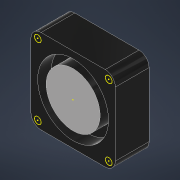
# Autodesk Inventor part: fan
Saved by Autodesk Inventor 2021 (Build 250183000, 183)
## iProperties
Created: 2021-01-23
Part Number: fan
Material: Polyethylene, Low Density
Document SubType Name: Modeling
Designer: User
Density: 0.894 g/cm^3
Appearance: Smooth - Black
Author: User
Autodesk Inventor part; units mm, degrees
ref_plane "YZ Plane" through (0, 0, 0) normal (1, 0, 0) x (0, 1, 0)
ref_plane "XZ Plane" through (0, 0, 0) normal (0, 1, 0) x (-1, 0, 0)
ref_plane "XY Plane" through (0, 0, 0) normal (0, 0, 1) x (1, 0, 0)
sketch "Sketch1" plane through (0, 0, 0) normal (0, 0, 1) x (1, 0, 0)
  circle A0 centre (9.5, 9.5) radius 1 projected
  arc A1 (12.2, 7.5) -> (12.5, 7.8) centre (12.2, 7.8) ccw projected
  line L0 (12.5, 7.8) -> (12.5, 12.2) projected
  arc A2 (12.5, 12.2) -> (12.2, 12.5) centre (12.2, 12.2) ccw projected
  line L1 (12.2, 12.5) -> (7.8, 12.5) projected
  arc A3 (7.8, 12.5) -> (7.5, 12.2) centre (7.8, 12.2) ccw projected
  line L2 (7.5, 12.2) -> (7.5, 7.8) projected
  arc A4 (7.5, 7.8) -> (7.8, 7.5) centre (7.8, 7.8) ccw projected
  line L3 (7.8, 7.5) -> (12.2, 7.5) projected
  circle A5 centre (9.5, -9.5) radius 1 projected
  arc A6 (12.5, -7.8) -> (12.2, -7.5) centre (12.2, -7.8) ccw projected
  line L4 (12.2, -7.5) -> (7.8, -7.5) projected
  arc A7 (7.8, -7.5) -> (7.5, -7.8) centre (7.8, -7.8) ccw projected
  line L5 (7.5, -7.8) -> (7.5, -12.2) projected
  arc A8 (7.5, -12.2) -> (7.8, -12.5) centre (7.8, -12.2) ccw projected
  line L6 (7.8, -12.5) -> (12.2, -12.5) projected
  arc A9 (12.2, -12.5) -> (12.5, -12.2) centre (12.2, -12.2) ccw projected
  line L7 (12.5, -12.2) -> (12.5, -7.8) projected
  circle A10 centre (-9.5, -9.5) radius 1 projected
  arc A11 (-12.2, -7.5) -> (-12.5, -7.8) centre (-12.2, -7.8) ccw projected
  line L8 (-12.5, -7.8) -> (-12.5, -12.2) projected
  arc A12 (-12.5, -12.2) -> (-12.2, -12.5) centre (-12.2, -12.2) ccw projected
  line L9 (-12.2, -12.5) -> (-7.8, -12.5) projected
  arc A13 (-7.8, -12.5) -> (-7.5, -12.2) centre (-7.8, -12.2) ccw projected
  line L10 (-7.5, -12.2) -> (-7.5, -7.8) projected
  arc A14 (-7.5, -7.8) -> (-7.8, -7.5) centre (-7.8, -7.8) ccw projected
  line L11 (-7.8, -7.5) -> (-12.2, -7.5) projected
  circle A15 centre (-9.5, 9.5) radius 1 projected
  arc A16 (-12.5, 7.8) -> (-12.2, 7.5) centre (-12.2, 7.8) ccw projected
  line L12 (-12.2, 7.5) -> (-7.8, 7.5) projected
  arc A17 (-7.8, 7.5) -> (-7.5, 7.8) centre (-7.8, 7.8) ccw projected
  line L13 (-7.5, 7.8) -> (-7.5, 12.2) projected
  arc A18 (-7.5, 12.2) -> (-7.8, 12.5) centre (-7.8, 12.2) ccw projected
  line L14 (-7.8, 12.5) -> (-12.2, 12.5) projected
  arc A19 (-12.2, 12.5) -> (-12.5, 12.2) centre (-12.2, 12.2) ccw projected
  line L15 (-12.5, 12.2) -> (-12.5, 7.8) projected
  line L16 (9.5, 12.5) -> (-9.5, 12.5)
  line L17 (-12.5, 9.5) -> (-12.5, -9.5)
  line L18 (-9.5, -12.5) -> (9.5, -12.5)
  line L19 (12.5, -9.5) -> (12.5, 9.5)
  line L20 (12.5, 12.5) -> (-12.5, -12.5) construction
  line L21 (-12.5, 12.5) -> (12.5, -12.5) construction
  arc A20 (12.5, 9.5) -> (9.5, 12.5) centre (9.5, 9.5) ccw
  arc A21 (-9.5, 12.5) -> (-12.5, 9.5) centre (-9.5, 9.5) ccw
  arc A22 (-12.5, -9.5) -> (-9.5, -12.5) centre (-9.5, -9.5) ccw
  arc A23 (9.5, -12.5) -> (12.5, -9.5) centre (9.5, -9.5) ccw
  point P0 (0, 0)
  point P1 (0, 0)
  point P2 (-9.5, 12.5)
  point P3 (-12.5, -9.5)
  point P4 (-12.5, -9.5)
  dimension "d0" = 25
  dimension "d1" = 25
  dimension "d2" = 3
  constraints: 12 end point, 8 point on circle, 8 point on line, 8 tangent, 4 centre point, 3 equal radius, 2 midpoint, 2 parallel, 1 horizontal, 1 horizontal alignment, 1 perpendicular, 1 vertical alignment
  measures "d0" distance of L21.end L20.end
  measures "d1" distance of L20.end L21.start
  measures "d2" radius of A20
extrude "Extrusion1" add sketch "Sketch1" along normal blind 10 contours L3 A4 L2 A3 L1 A20 L0 A1 | A1 L19 A6 L4 A7 L5 A8 L18 A13 L10 A14 L11 A11 L17 A16 L12 A17 L13 A18 L16 A3 L2 A4 L3 | L7 A23 L6 A8 L5 A7 L4 A6 | A18 L13 A17 L12 A16 L15 A21 L14 | L9 A22 L8 A11 L11 A14 L10 A13
sketch "Sketch2" plane through (0, 0, 10) normal (0, 0, 1) x (1, 0, 0)
  circle A0 centre (0, 0) radius 10.5
  dimension "d5" = 21
  constraints: 1 centre point, 1 coincident
  measures "d5" diameter of A0
extrude "Extrusion2" cut sketch "Sketch2" against normal blind 4
sketch "Sketch3" plane through (0, 0, 6) normal (0, 0, 1) x (1, 0, 0)
  circle A0 centre (0, 0) radius 8
  dimension "d8" = 16
  constraints: 1 centre point, 1 coincident
  measures "d8" diameter of A0
extrude "Extrusion3" add sketch "Sketch3" along normal up to surface (4 mm away)
sketch "Sketch4" plane through (0, 0, 10) normal (0, 0, 1) x (1, 0, 0)
  circle A0 centre (9.5, -9.5) radius 1 projected
  circle A1 centre (-9.5, -9.5) radius 1 projected
  circle A2 centre (-9.5, 9.5) radius 1 projected
  circle A3 centre (9.5, 9.5) radius 1 projected
  circle A4 centre (9.5, -9.5) radius 2.5
  line L0 (-9.5, -12.5) -> (9.5, -12.5) projected
  line L1 (12.5, -9.5) -> (12.5, 9.5) projected
  circle A5 centre (-9.5, -9.5) radius 2.5
  circle A6 centre (9.5, 9.5) radius 2.5
  circle A7 centre (-9.5, 9.5) radius 2.5
  point P0 (0, 0)
  dimension "d11" = 5
  dimension "d12" = 19
  dimension "d13" = 19
  dimension "d16" = 19
  dimension "d19" = 19
  constraints: 4 centre point, 1 coincident, 1 horizontal, 1 vertical, 6 other
  measures "d11" diameter of A4
  measures "d12" distance of A1.centre A0.centre
  measures "d13" distance of A3.centre A0.centre
  measures "d16" distance of A4.centre A5.centre
  measures "d19" distance of A4.centre A6.centre
extrude "Extrusion4" cut sketch "Sketch4" against normal blind 1 contours A0 | A1 | A2 | A3 | A4 | A5 | A6 | A7
equation "\"d16\" = d12"
equation "\"d19\" = d13"
body "Solid1"
